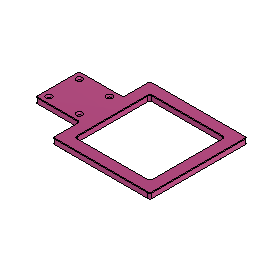
plate (Autodesk Fusion 360 design; units mm, degrees)
Autodesk Fusion 360 part; units mm, degrees
sketch "Cuadrado 100x100" plane through (0, 0, 0) normal (0, 0, 1) x (1, 0, 0)
  line L0 (50, -50) -> (-50, -50)
  line L1 (-50, -50) -> (-50, 50)
  line L2 (-50, 50) -> (50, 50)
  line L3 (50, 50) -> (50, -50)
  line L4 (50, -50) -> (-50, 50) construction
  line L5 (-50, -50) -> (50, 50) construction
  dimension "d1" = 100
  constraint perpendicular L0 L1
  constraint parallel L0 L2
  constraint parallel L1 L3
  constraint horizontal L0
  constraint coincident L4 origin
  constraint coincident L5 origin
  constraint equal L1 L2
  measures "d1" distance of L0.end L1.end
sketch "Sketch1" plane through (0, 0, 0) normal (0, 0, 1) x (1, 0, 0) in component "plate"
  line L0 (22.5, 22.5) -> (-22.5, 22.5)
  line L1 (-22.5, 22.5) -> (-22.5, -22.5)
  line L2 (-22.5, -22.5) -> (22.5, -22.5)
  line L3 (22.5, -22.5) -> (22.5, 22.5)
  line L4 (22.5, 22.5) -> (-22.5, -22.5) construction
  line L5 (-22.5, 22.5) -> (22.5, -22.5) construction
  line L6 (15.5, 15.5) -> (-15.5, 15.5)
  line L7 (-15.5, 15.5) -> (-15.5, -15.5)
  line L8 (-15.5, -15.5) -> (15.5, -15.5)
  line L9 (15.5, -15.5) -> (15.5, 15.5)
  line L10 (122.5, -50) -> (22.5, -50)
  line L11 (22.5, -50) -> (22.5, 50)
  line L12 (22.5, 50) -> (122.5, 50)
  line L13 (122.5, 50) -> (122.5, -50)
  line L14 (122.5, -50) -> (22.5, 50) construction
  line L15 (22.5, -50) -> (122.5, 50) construction
  line L16 (110.7039, 38.2039) -> (34.2961, 38.2039)
  line L17 (34.2961, 38.2039) -> (34.2961, -38.2039)
  line L18 (34.2961, -38.2039) -> (110.7039, -38.2039)
  line L19 (110.7039, -38.2039) -> (110.7039, 38.2039)
  line L20 (72.5, 0) -> (22.5, 0) construction
  point P0 (72.5, 0)
  point P1 (72.5, 0)
  dimension "d59" = 45
  dimension "d60" = 31
  dimension "d62" = 100
  constraint perpendicular L0 L1
  constraint parallel L0 L2
  constraint parallel L1 L3
  constraint horizontal L0
  constraint coincident L4 origin
  constraint coincident L5 origin
  constraint horizontal L6
  constraint perpendicular L10 L11
  constraint parallel L10 L12
  constraint parallel L11 L13
  constraint horizontal L10
  constraint coincident L14 P1
  constraint coincident L15 P1
  constraint equal L12 L13
  constraint equal L0 L1
  constraint coincident P1 P0
  constraint horizontal L16
  constraint coincident L10.end L11.start
  constraint midpoint L3 L20.end
  constraint horizontal L20
  constraint collinear L3 L11
  measures "d59" distance of L0.start L0.end
  measures "d60" distance of L6.start L6.end
  measures "d62" distance of L11.end L12.end
extrude "Extrude1" add sketch "Sketch1" against normal blind 6 contours L0 L1 L2 L3 L11 | L3 L10 L11 L12 L13 | L6 L7 L8 L9 in component "plate"
fillet "Fillet1" radius 2 14 edges at (-22.5, 22.5, -3) (-22.5, -22.5, -3) (22.5, 22.5, -3) (22.5, 50, -3) (122.5, 50, -3) (122.5, -50, -3) (22.5, -22.5, -3) (22.5, -50, -3) (22.5, -22.5, -3) (22.5, -50, -3) (34.2961, 38.2039, -3) (110.7039, 38.2039, -3) (110.7039, -38.2039, -3) (34.2961, -38.2039, -3) in component "plate"
chamfer "Chamfer1" distance 0.5 angle 45 48 edges at (122.5, 0, 0) (121.9142, -49.4142, 0) (72.5, -50, 0) (23.0858, -49.4142, 0) (22.5, -36.25, 0) (21.9142, -23.0858, 0) (0, -22.5, 0) (-21.9142, -21.9142, 0) (-22.5, 0, 0) (-21.9142, 21.9142, 0) (0, 22.5, 0) (21.9142, 23.0858, 0) (22.5, 36.25, 0) (23.0858, 49.4142, 0) (72.5, 50, 0) (121.9142, 49.4142, 0) (122.5, 0, -6) (121.9142, 49.4142, -6) (72.5, 50, -6) (23.0858, 49.4142, -6) (22.5, 36.25, -6) (21.9142, 23.0858, -6) (0, 22.5, -6) (-21.9142, 21.9142, -6) (-22.5, 0, -6) (-21.9142, -21.9142, -6) (0, -22.5, -6) (21.9142, -23.0858, -6) (22.5, -36.25, -6) (23.0858, -49.4142, -6) (72.5, -50, -6) (121.9142, -49.4142, -6) (34.8819, 37.6181, -6) (34.2961, 0, -6) (34.8819, -37.6181, -6) (72.5, -38.2039, -6) (110.1181, -37.6181, -6) (110.7039, 0, -6) (110.1181, 37.6181, -6) (72.5, 38.2039, -6) (110.1181, 37.6181, 0) (110.7039, 0, 0) (110.1181, -37.6181, 0) (72.5, -38.2039, 0) (34.8819, -37.6181, 0) (34.2961, 0, 0) (34.8819, 37.6181, 0) (72.5, 38.2039, 0) in component "plate"
hole "Hole1" at (15.5, 15.5, 0) at (-15.5, 15.5, 0) at (-15.5, -15.5, 0) at (15.5, -15.5, 0) direction (0, 0, -1) diameter 3 end through all countersink diameter 6 countersink angle 90 in component "plate"
component "plate" placed x (1, 0, 0) y (0, 1, 0) z (0, 0, 1) at (0, 0, 0)
equation "offsetI3dDiam = 0.2 mm"
equation "offsetI3dRad = offsetI3dDiam / 2"
